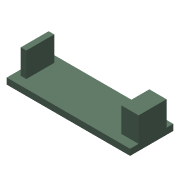
# Autodesk Inventor part: 00_LM286
Saved by Autodesk Inventor 2019.4 (Build 234330000, 330)
## iProperties
Created: 2021-06-01
Part Number: 00_LM286
Material: Generic
Document SubType Name: Modeling
Designer: diederichbenedict
Density: 1 g/cm^3
Appearance: Rubber - Green
Author: diederichbenedict
Autodesk Inventor part; units mm, degrees
ref_plane "YZ Plane" through (0, 0, 0) normal (1, 0, 0) x (0, 1, 0)
ref_plane "XZ Plane" through (0, 0, 0) normal (0, 1, 0) x (-1, 0, 0)
ref_plane "XY Plane" through (0, 0, 0) normal (0, 0, 1) x (1, 0, 0)
sketch "Sketch1" plane through (0, 0, 0) normal (0, 1, 0) x (-1, 0, 0)
  line L0 (0, 0) -> (40, 0)
  line L1 (40, 0) -> (40, 14)
  line L2 (40, 14) -> (0, 14)
  line L3 (0, 14) -> (0, 0)
  dimension "d0" = 40
  dimension "d1" = 14
  constraints: 8 end point, 2 parallel, 1 horizontal, 1 perpendicular
  measures "d0" distance of L2.end L1.end
  measures "d1" distance of L1.end L0.end
extrude "Extrusion1" add sketch "Sketch1" along normal blind 2
sketch "Sketch2" plane through (0, 2, 0) normal (0, 1, 0) x (1, 0, 0)
  line L0 (0, -14) -> (0, 0) projected
  line L1 (0, -11.242) -> (-5.5713, -11.242)
  line L2 (-5.5713, -11.242) -> (-5.5713, -2.1887)
  line L3 (-5.5713, -2.1887) -> (0, -2.1887)
  line L4 (0, -2.1887) -> (0, -11.242)
  line L5 (-38.2029, -11.242) -> (-36.4121, -11.242)
  line L6 (-36.4121, -11.242) -> (-36.4121, -2.1887)
  line L7 (-36.4121, -2.1887) -> (-38.2029, -2.1887)
  line L8 (-38.2029, -2.1887) -> (-38.2029, -11.242)
  constraints: 16 end point, 4 parallel, 3 point on line, 2 horizontal, 2 perpendicular
extrude "Extrusion2" add sketch "Sketch2" along normal blind 8
body "Solid1"
